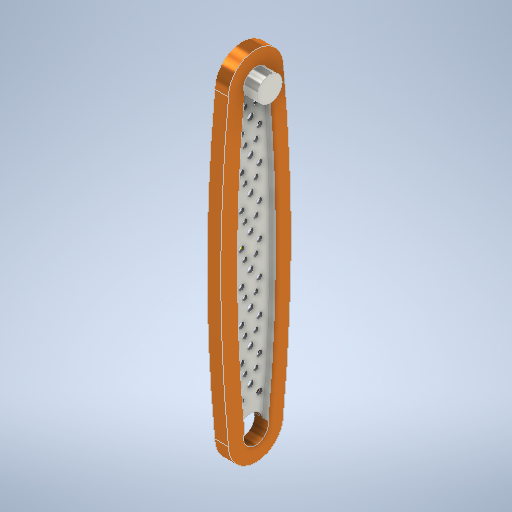
# Autodesk Inventor part: odnoga1
Saved by Autodesk Inventor 2025 (Build 290162000, 162)
## iProperties
Created: 2024-04-20
Part Number: odnoga1
Material: Generic
Document SubType Name: Modeling
Designer: joann
Density: 1 g/cm^3
Appearance: Default
Author: joann
Autodesk Inventor part; units mm, degrees
ref_plane "YZ Plane" through (0, 0, 0) normal (1, 0, 0) x (0, 1, 0)
ref_plane "XZ Plane" through (0, 0, 0) normal (0, 1, 0) x (-1, 0, 0)
ref_plane "XY Plane" through (0, 0, 0) normal (0, 0, 1) x (1, 0, 0)
sketch "Sketch1" plane through (0, 0, 0) normal (1, 0, 0) x (0, 1, 0)
  line L0 (-91, 0) -> (91, 0) projected
  circle A0 centre (55, 0) radius 10
  circle A1 centre (-55, 0) radius 10
  circle A2 centre (55, 0) radius 4.5
  circle A3 centre (-55, 0) radius 4.5
  line L1 (0, -755.8217) -> (0, 755.8217) projected
  arc A4 (55, 10) -> (-55, 10) centre (0, -534.3421) ccw
  arc A5 (-55, -10) -> (55, -10) centre (0, 534.3421) ccw
  arc A6 (55, 4.5) -> (-55, 4.5) centre (0, -539.8726) ccw
  arc A7 (-55, -4.5) -> (55, -4.5) centre (0, 539.8726) ccw
  point P0 (0, 0)
  point P1 (0, -12.7715)
  point P2 (0, 12.7715)
  dimension "d2" = 20
  dimension "d4" = 9
  dimension "d5" = 9
  dimension "d6" = 110
  dimension "d7" = 547.1136
  dimension "d8" = 110
  dimension "d9" = 547.1136
  dimension "d10" = 20
  dimension "d11" = 25.5431
  dimension "d16" = 547.144
  dimension "d17" = 547.144
  constraints: 18 point on circle, 8 centre point, 4 coincident, 2 horizontal alignment, 1 symmetric about line, 1 other
  measures "d2" diameter of A0
  measures "d4" diameter of A2
  measures "d5" diameter of A3
  measures "d6" distance of A1.end A0.end
  measures "d7" radius of A5
  measures "d8" distance of A1.centre A0.centre
  measures "d9" radius of A4
  measures "d10" diameter of A1
  measures "d11" distance of point (0, -12.772) point (0, 12.772)
  measures "d16" radius of A6
  measures "d17" radius of A7
extrude "Extrusion1" add sketch "Sketch1" along normal mid plane 5 contours A3 A6 A1 L0 | L0 A1 A7 A3 | A1 A6 L1 L0 | L0 L1 A7 A1 | A3 A7 A1 L0 | L0 A1 A6 A3 | L1 A6 A0 L0 | L0 A0 A7 L1 | A1 A4 L1 A6 | A7 L1 A5 A1 | A0 A6 A2 L0 | L0 A2 A7 A0 | A7 A0 A5 L1 | L1 A4 A0 A6 | A2 L0 | L0 A2 | A0 L0 A2 A6 | A7 A2 L0 A0
sketch "Sketch2" plane through (-2.5, 0, 0) normal (-1, 0, 0) x (0, 0, 1)
  point P0 (0, 0)
sketch "Sketch3" plane through (2.5, 0, 0) normal (1, 0, 0) x (0, 0, -1)
  circle A0 centre (0, 55) radius 4.5
  circle A1 centre (0, -55) radius 4.5 projected
  line L0 (17.8801, 0) -> (-17.8801, 0) projected
  point P0 (0, 0)
  constraints: 1 centre point, 1 equal radius, 1 other
extrude "Extrusion2" add sketch "Sketch3" along normal blind 5 contours A0
sketch "Sketch4" plane through (2.5, 0, 0) normal (1, 0, 0) x (0, 0, -1)
  circle A0 centre (0, 55) radius 4.5 projected
  circle A1 centre (0, -55) radius 4.5 projected
  arc A2 (-4.1071, 53.1611) -> (-4.1071, -53.1611) centre (540.4481, 0) ccw
  arc A3 (4.0879, -56.8812) -> (4.0879, 56.8812) centre (-540.0914, 0) ccw
  arc A4 (4.0879, -56.8812) -> (4.0879, 56.8812) centre (-540.0914, 0) ccw
  arc A5 (4.0879, -56.8812) -> (4.0879, 56.8812) centre (-540.0914, 0) ccw
  arc A6 (-4.1071, 53.1611) -> (-4.1071, -53.1611) centre (540.4481, 0) ccw
  circle A7 centre (0, 55) radius 4.5
  point P0 (0, 0)
  point P1 (4.3832, -53.9815)
  point P2 (4.3832, 53.9815)
  dimension "d18" = 547.144
  dimension "d19" = 547.144
  constraints: 14 point on circle, 6 centre point, 5 concentric
  measures "d18" radius of A2
  measures "d19" radius of A3
extrude "Extrusion3" cut sketch "Sketch4" against normal blind 2 contours A3 A1 A2 A0
sketch "Sketch5" plane through (2.5, 0, 0) normal (1, 0, 0) x (0, 0, -1)
  circle A0 centre (0, 55) radius 4.5 projected
  circle A1 centre (0, -55) radius 4.5 projected
  arc A2 (-3.2318, 51.8686) -> (-3.2318, -51.8686) centre (541.4481, 0) ccw
  arc A3 (3.5532, -52.2387) -> (3.5532, 52.2387) centre (-541.0914, 0) ccw
  arc A4 (4.3832, -53.9815) -> (4.3832, 53.9815) centre (-540.0914, 0) ccw projected
  arc A5 (-4.1071, 53.1611) -> (-4.1071, -53.1611) centre (540.4481, 0) ccw projected
  circle A6 centre (-2, 46.7386) radius 1
  circle A7 centre (2, 46.7386) radius 1
  line L0 (0, -91) -> (0, 91) projected
  circle A8 centre (0, 42.7386) radius 1.25
  circle A9 centre (3.25, 38.7386) radius 1.1
  circle A10 centre (-3.25, 38.7386) radius 1.1
  point P0 (0, 0)
  point P1 (-5.6959, 0)
  point P2 (6.0526, 0)
  point P3 (7.0526, 0)
  point P4 (-6.6959, 0)
  dimension "d26" = 1
  dimension "d27" = 1
  dimension "d28" = 547.144
  dimension "d29" = 547.144
  dimension "d30" = 4
  dimension "d31" = 2
  dimension "d32" = 2
  dimension "d33" = 2.5
  dimension "d35" = 3
  dimension "d41" = 2.2
  dimension "d42" = 2.2
  dimension "d44" = 8
  dimension "d45" = 6.5
  dimension "d46" = 4
  constraints: 12 point on circle, 7 centre point, 2 horizontal alignment, 2 symmetric about line, 1 point on line
  measures "d26" distance of point (7.053, 0) point (6.053, 0)
  measures "d27" distance of point (-6.696, 0) point (-5.696, 0)
  measures "d28" radius of A3
  measures "d29" radius of A2
  measures "d30" distance of A7.centre A6.centre
  measures "d31" diameter of A6
  measures "d32" diameter of A7
  measures "d33" diameter of A8
  measures "d41" diameter of A9
  measures "d42" diameter of A10
  measures "d44" vertical distance of A7.centre A9.centre
  measures "d45" distance of A9.centre A10.centre
  measures "d46" vertical distance of A8.centre A6.centre
extrude "Extrusion4" cut sketch "Sketch5" against normal through all contours A10 A2 | A2 A10 | A8 L0 | L0 A8 | A6 | A7 | A9
pattern_linear "Rectangular Pattern1" count 8 spacing 12 along (0, -1, 0) of "Extrusion4"
sketch "Sketch6" plane through (-2.5, 0, 0) normal (-1, 0, 0) x (0, 0, 1)
  arc A0 (-4.3832, 53.9815) -> (4.1071, 53.1611) centre (0, 55) ccw projected
  arc A1 (-4.3832, 53.9815) -> (-4.3832, -53.9815) centre (540.0914, 0) ccw projected
  arc A2 (-4.3832, 53.9815) -> (-4.3832, -53.9815) centre (540.0914, 0) ccw
  arc A3 (4.1071, -53.1611) -> (4.1071, 53.1611) centre (-540.4481, 0) ccw projected
  arc A4 (4.1071, -53.1611) -> (4.1071, 53.1611) centre (-540.4481, 0) ccw
  circle A5 centre (0, -55) radius 4.5
  circle A6 centre (0, -55) radius 4.5 projected
  arc A7 (10, -55) -> (10, 55) centre (-534.3421, 0) ccw projected
  arc A8 (-10, 55) -> (-10, -55) centre (534.3421, 0) ccw projected
  point P0 (0, 0)
  point P1 (12.7715, 0)
  point P2 (6.6959, 0)
  point P3 (-12.7715, 0)
  point P4 (-7.0526, 0)
  point P5 (6.6959, 0)
  point P6 (-4.3832, -53.9815)
  dimension "d50" = 9
  dimension "d47" = 6.0757
  dimension "d48" = 5.7189
  dimension "d51" = 547.144
  dimension "d52" = 4.5
  dimension "d53" = 547.144
  constraints: 9 point on circle, 2 centre point, 4 other
  measures "d47" distance of point (12.772, 0) point (6.696, 0)
  measures "d48" distance of point (-12.772, 0) point (-7.053, 0)
  measures "d51" radius of A3
  measures "d52" radius of A0
  measures "d53" radius of A2
extrude "Extrusion5" cut sketch "Sketch6" against normal blind 2 contours A0 A3 A5 A1
body "Solid1"
